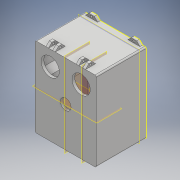
# Autodesk Inventor part: Base
Saved by Autodesk Inventor 2017 (Build 210142000, 142)
## iProperties
Created: 2017-05-28
Part Number: Base
Material: Generic
Document SubType Name: Modeling
Designer: William
Density: 1 g/cm^3
Appearance: Default
Author: William
Autodesk Inventor part; units mm, degrees
ref_plane "YZ Plane" through (0, 0, 0) normal (1, 0, 0) x (0, 1, 0)
ref_plane "XZ Plane" through (0, 0, 0) normal (0, 1, 0) x (-1, 0, 0)
ref_plane "XY Plane" through (0, 0, 0) normal (0, 0, 1) x (1, 0, 0)
sketch "Sketch1" plane through (0, 0, 0) normal (0, 1, 0) x (-1, 0, 0)
  line L0 (0, 0) -> (47, 0) construction
  line L1 (47, 0) -> (47, -100) construction
  line L2 (47, -100) -> (0, -100) construction
  line L3 (0, -100) -> (0, 0) construction
  circle A0 centre (4, -4) radius 1.6 construction
  circle A1 centre (43, -4) radius 1.6 construction
  circle A2 centre (43, -96) radius 1.729 construction
  line L4 (23.5, 0) -> (23.5, -100) construction
  line L5 (23.5, -13) -> (18.5, -13) construction
  line L6 (18.5, -13) -> (0.5, -13) construction
  circle A3 centre (0.5, -13) radius 13.5 construction
  line L7 (23.5, -13) -> (46.5, -13) construction
  circle A4 centre (46.5, -13) radius 13.5 construction
  circle A5 centre (46.5, -13) radius 13.5
  circle A6 centre (0.5, -13) radius 13.5
  circle A7 centre (23.5, -50) radius 8
  line L8 (65, 5.5) -> (-18, 5.5)
  line L9 (-18, 5.5) -> (-18, -105)
  line L10 (-18, -105) -> (65, -105)
  line L11 (65, -105) -> (65, 5.5)
  dimension "d0" = 47
  dimension "d1" = 100
  dimension "d2" = 3.2
  dimension "d3" = 4
  dimension "d4" = 4
  dimension "d5" = 4
  dimension "d6" = 43
  dimension "d7" = 3.2
  dimension "d8" = 43
  dimension "d9" = 96
  dimension "d11" = 23.5
  dimension "d12" = 5
  dimension "d13" = 13
  dimension "d14" = 18
  dimension "d15" = 27
  dimension "d16" = 23
  dimension "d17" = 27
  dimension "d18" = 16
  dimension "d19" = 50
  dimension "d20" = 5
  dimension "d21" = 5
  dimension "d22" = 5
  dimension "d23" = 5
  constraints: 24 end point, 8 centre point, 4 coincident, 4 horizontal, 4 parallel, 4 perpendicular, 3 midpoint, 2 concentric, 1 point on line
  measures "d0" distance of L1.end L2.end
  measures "d1" distance of L0.end L1.end
  measures "d2" diameter of A0
  measures "d3" distance from line of L0 A0.centre
  measures "d4" distance from line of L3 A0.centre
  measures "d5" distance from line of L0 A1.centre
  measures "d6" distance from line of L3 A1.centre
  measures "d7" diameter of A1
  measures "d8" distance from line of L3 A2.centre
  measures "d9" distance from line of L0 A2.centre
  measures "d11" distance between parallel lines of L3 L4
  measures "d12" distance of L5.start L5.end
  measures "d13" distance between parallel lines of L0 L5
  measures "d14" distance of L5.end L6.end
  measures "d15" diameter of A3
  measures "d16" distance of L5.start L7.end
  measures "d17" diameter of A4
  measures "d18" diameter of A7
  measures "d19" distance of L4.start A7.centre
  measures "d20" distance edge to line of A4 L11
  measures "d21" distance edge to line of A6 L9
  measures "d22" distance edge to line of A4 L8
  measures "d23" distance between parallel lines of L2 L10
extrude "Extrusion1" add sketch "Sketch1" along normal blind 4
sketch "Sketch3" plane through (0, 0, 0) normal (0, -1, 0) x (1, 0, 0)
  line L0 (22, -109) -> (-69, -109)
  line L1 (-69, -109) -> (-69, 9.5)
  line L2 (-69, 9.5) -> (22, 9.5)
  line L3 (22, 9.5) -> (22, -109)
  line L4 (-65, 5.5) -> (18, 5.5) projected
  line L5 (18, 5.5) -> (18, -105) projected
  line L6 (-65, 5.5) -> (18, 5.5)
  line L7 (18, 5.5) -> (18, -105)
  line L8 (18, -105) -> (-65, -105)
  line L9 (-65, -105) -> (-65, 5.5)
  point P0 (0, 0)
  dimension "d30" = 4
  dimension "d31" = 4
  dimension "d32" = 4
  dimension "d33" = 4
  constraints: 16 end point, 4 parallel, 2 horizontal, 2 perpendicular
  measures "d30" distance between parallel lines of L3 L5
  measures "d31" distance between parallel lines of L2 L4
  measures "d32" distance between parallel lines of L1 L9
  measures "d33" distance between parallel lines of L0 L8
extrude "Extrusion2" add sketch "Sketch3" against normal blind 74
sketch "Sketch4" plane through (0, 74, 0) normal (0, 1, 0) x (1, 0, 0)
  line L0 (-68, -8.5) -> (21, -8.5)
  line L1 (21, -8.5) -> (21, 108)
  line L2 (21, 108) -> (-68, 108)
  line L3 (-68, 108) -> (-68, -8.5)
  line L4 (19, 106) -> (-66, 106)
  line L5 (-66, 106) -> (-66, -6.5)
  line L6 (-66, -6.5) -> (19, -6.5)
  line L7 (19, -6.5) -> (19, 106)
  line L8 (-69, -9.5) -> (22, -9.5) projected
  line L9 (22, -9.5) -> (22, 109) projected
  line L10 (22, 109) -> (-69, 109) projected
  line L11 (-69, 109) -> (-69, -9.5) projected
  point P0 (0, 0)
  dimension "d36" = 1
  dimension "d37" = 2
  dimension "d38" = 1
  dimension "d39" = 2
  dimension "d40" = 1
  dimension "d41" = 2
  dimension "d42" = 1
  dimension "d43" = 2
  constraints: 16 end point, 4 parallel, 2 horizontal, 2 perpendicular
  measures "d36" distance between parallel lines of L8 L0
  measures "d37" distance between parallel lines of L0 L6
  measures "d38" distance between parallel lines of L9 L1
  measures "d39" distance between parallel lines of L1 L7
  measures "d40" distance between parallel lines of L10 L2
  measures "d41" distance between parallel lines of L2 L4
  measures "d42" distance between parallel lines of L11 L3
  measures "d43" distance between parallel lines of L3 L5
extrude "Extrusion3" cut sketch "Sketch4" against normal blind 4 contours L3 L2 L1 L0
fillet "Fillet1" radius 2 16 edges at (-69, 37, 9.5) (-68, 72, 8.5) (-66, 72, 6.5) (-65, 39, 5.5) (19, 72, 6.5) (21, 72, 8.5) (18, 39, 5.5) (22, 37, 9.5) (22, 37, -109) (19, 72, -106) (18, 39, -105) (21, 72, -108) (-65, 39, -105) (-68, 72, -108) (-69, 37, -109) (-66, 72, -106)
ref_plane "Work Plane1" through (0, 64, 0) normal (0, 1, 0) x (1, 0, 0)
sketch "Sketch6" plane through (0, 64, 0) normal (0, 1, 0) x (1, 0, 0)
  line L0 (0, 0) -> (-47, 0) construction
  line L1 (-47, 0) -> (-47, 100) construction
  line L2 (-47, 100) -> (0, 100) construction
  line L3 (0, 100) -> (0, 0) construction
  circle A0 centre (-4, 4) radius 1.6 construction
  circle A1 centre (-42.7634, 4) radius 1.6 construction
  line L4 (18, -3.5) -> (18, 103) projected
  line L5 (10, 34.5) -> (10, 54.5)
  line L6 (16, -5.5) -> (-63, -5.5) projected
  circle A2 centre (14, 38.5) radius 1.6
  circle A3 centre (14, 50.5) radius 1.6
  line L7 (10, 34.5) -> (18, 26.5)
  line L8 (10, 34.5) -> (21.3137, 34.5) construction
  line L9 (10, 54.5) -> (18, 62.5)
  line L10 (10, 54.5) -> (21.3137, 54.5) construction
  line L11 (18, 26.5) -> (18, 62.5)
  line L12 (-57, 34.5) -> (-57, 54.5)
  line L13 (-57, 34.5) -> (-37, 34.5) construction
  line L14 (-65, 103) -> (-65, -3.5) projected
  line L15 (-57, 34.5) -> (-65, 26.5)
  line L16 (-57, 34.5) -> (-45.6863, 34.5) construction
  line L17 (-57, 54.5) -> (-65, 62.5)
  line L18 (-57, 54.5) -> (-45.6863, 54.5) construction
  line L19 (-65, 62.5) -> (-65, 26.5)
  circle A4 centre (-61, 38.5) radius 1.6
  circle A5 centre (-61, 50.5) radius 1.6
  dimension "d48" = 47
  dimension "d49" = 100
  dimension "d50" = 3.2
  dimension "d51" = 4
  dimension "d52" = 4
  dimension "d53" = 3.2
  dimension "d55" = 20
  dimension "d57" = 3.2
  dimension "d58" = 3.2
  dimension "d61" = 4
  dimension "d62" = 4
  dimension "d63" = 45
  dimension "d64" = 45
  dimension "d65" = 20
  dimension "d66" = 90
  dimension "d67" = 8
  dimension "d68" = 135
  dimension "d69" = 135
  dimension "d70" = 3.2
  dimension "d71" = 3.2
  dimension "d100" = 12
  dimension "d101" = 0
  dimension "d102" = 4
  dimension "d103" = 12
  constraints: 34 end point, 6 centre point, 6 horizontal, 5 equal length, 4 point on line, 2 collinear, 2 parallel, 1 perpendicular, 1 vertical
  measures "d48" distance of L1.end L2.end
  measures "d49" distance of L0.end L1.end
  measures "d50" diameter of A0
  measures "d51" distance from line of L3 A0.centre
  measures "d52" distance from line of L0 A0.centre
  measures "d53" diameter of A1
  measures "d55" distance of L5.start L5.end
  measures "d57" diameter of A2
  measures "d58" diameter of A3
  measures "d61" distance from line of L5 A2.centre
  measures "d62" distance from line of L5 A3.centre
  measures "d63" angle of L7 L8
  measures "d64" angle of L10 L9
  measures "d65" distance of L12.start L12.end
  measures "d66" angle of L13 L12
  measures "d67" distance between parallel lines of L14 L12
  measures "d68" angle of L15 L16
  measures "d69" angle of L18 L17
  measures "d70" diameter of A4
  measures "d71" diameter of A5
  measures "d100" distance of A4.centre A5.centre
  measures "d101" vertical distance of A3.centre A5.centre
  measures "d102" distance from line of L8 A2.centre
  measures "d103" distance of A2.centre A3.centre
extrude "Extrusion4" add sketch "Sketch6" against normal up to next
sketch "Sketch8" plane through (0, 74, 0) normal (0, 1, 0) x (1, 0, 0)
  line L0 (-51, -14.5) -> (-59, -14.5)
  line L1 (-69, 107) -> (-69, -7.5) projected
  line L2 (4, -14.5) -> (12, -14.5)
  line L3 (22, -7.5) -> (22, 107) projected
  line L4 (-59, -14.5) -> (-64, -9.5)
  line L5 (-59, -14.5) -> (-51.9289, -14.5) construction
  line L6 (-51, -14.5) -> (-46, -9.5)
  line L7 (-51, -14.5) -> (-43.9289, -14.5) construction
  line L8 (-46, -9.5) -> (-64, -9.5)
  line L9 (-67, -9.5) -> (20, -9.5) projected
  line L10 (4, -14.5) -> (-1, -9.5)
  line L11 (4, -14.5) -> (11.0711, -14.5) construction
  line L12 (12, -14.5) -> (17, -9.5)
  line L13 (12, -14.5) -> (19.0711, -14.5) construction
  line L14 (17, -9.5) -> (-1, -9.5)
  circle A0 centre (-55.4645, -12) radius 1.6
  circle A1 centre (8, -12) radius 1.6
  line L15 (20, 109) -> (-67, 109) projected
  line L16 (-51, 114) -> (-59, 114)
  line L17 (4, 114) -> (12, 114)
  line L18 (-51, 114) -> (-46, 109)
  line L19 (-51, 114) -> (-43.9289, 114) construction
  line L20 (-59, 114) -> (-64, 109)
  line L21 (-59, 114) -> (-51.9289, 114) construction
  line L22 (-64, 109) -> (-46, 109)
  line L23 (4, 114) -> (-1, 109)
  line L24 (4, 114) -> (11.0711, 114) construction
  line L25 (12, 114) -> (17, 109)
  line L26 (-1, 109) -> (17, 109)
  circle A2 centre (-55, 111.5) radius 1.6
  circle A3 centre (8, 111.5) radius 1.6
  point P0 (0, 0)
  dimension "d74" = 8
  dimension "d77" = 8
  dimension "d80" = 135
  dimension "d81" = 45
  dimension "d82" = 135
  dimension "d83" = 45
  dimension "d84" = 3.2
  dimension "d85" = 3.2
  dimension "d86" = 8
  dimension "d89" = 8
  dimension "d91" = 10
  dimension "d92" = 10
  dimension "d93" = 45
  dimension "d94" = 135
  dimension "d95" = 135
  dimension "d96" = 3.2
  dimension "d97" = 3.2
  constraints: 46 end point, 7 equal length, 7 horizontal, 6 point on line, 4 centre point, 4 collinear
  measures "d74" distance of L0.start L0.end
  measures "d77" distance of L2.end L2.start
  measures "d80" angle of L5 L4
  measures "d81" angle of L7 L6
  measures "d82" angle of L11 L10
  measures "d83" angle of L13 L12
  measures "d84" diameter of A0
  measures "d85" diameter of A1
  measures "d86" distance of L16.end L16.start
  measures "d89" distance of L17.start L17.end
  measures "d91" distance from line of L3 L17.end
  measures "d92" distance from line of L1 L16.end
  measures "d93" angle of L18 L19
  measures "d94" angle of L20 L21
  measures "d95" angle of L23 L24
  measures "d96" diameter of A2
  measures "d97" diameter of A3
extrude "Extrusion5" add sketch "Sketch8" against normal blind 4
sketch "Sketch9" plane through (0, 74, 0) normal (0, 1, 0) x (1, 0, 0)
  circle A0 centre (-55, 111.5) radius 1.6 projected
  circle A1 centre (-55.4645, -12) radius 1.6 projected
  circle A2 centre (8, -12) radius 1.6 projected
  circle A3 centre (8, 111.5) radius 1.6 projected
  arc A4 (-67, 109) -> (-69, 107) centre (-67, 107) ccw projected
  line L0 (-69, 107) -> (-69, -7.5) projected
  arc A5 (-69, -7.5) -> (-67, -9.5) centre (-67, -7.5) ccw projected
  line L1 (-67, -9.5) -> (-64, -9.5) projected
  line L2 (-59, -14.5) -> (-64, -9.5) projected
  line L3 (-51, -14.5) -> (-59, -14.5) projected
  line L4 (-46, -9.5) -> (-51, -14.5) projected
  line L5 (-46, -9.5) -> (-1, -9.5) projected
  line L6 (-1, -9.5) -> (4, -14.5) projected
  line L7 (4, -14.5) -> (12, -14.5) projected
  line L8 (12, -14.5) -> (17, -9.5) projected
  line L9 (17, -9.5) -> (20, -9.5) projected
  arc A6 (20, -9.5) -> (22, -7.5) centre (20, -7.5) ccw projected
  line L10 (22, -7.5) -> (22, 107) projected
  arc A7 (22, 107) -> (20, 109) centre (20, 107) ccw projected
  line L11 (20, 109) -> (17, 109) projected
  line L12 (17, 109) -> (12, 114) projected
  line L13 (12, 114) -> (4, 114) projected
  line L14 (4, 114) -> (-1, 109) projected
  line L15 (-1, 109) -> (-46, 109) projected
  line L16 (-46, 109) -> (-51, 114) projected
  line L17 (-51, 114) -> (-59, 114) projected
  line L18 (-59, 114) -> (-64, 109) projected
  line L19 (-64, 109) -> (-67, 109) projected
  line L20 (21, 106) -> (21, -6.5) projected
  arc A8 (19, -8.5) -> (21, -6.5) centre (19, -6.5) ccw projected
  line L21 (19, -8.5) -> (-66, -8.5) projected
  arc A9 (-68, -6.5) -> (-66, -8.5) centre (-66, -6.5) ccw projected
  line L22 (-68, -6.5) -> (-68, 106) projected
  arc A10 (-66, 108) -> (-68, 106) centre (-66, 106) ccw projected
  line L23 (-66, 108) -> (19, 108) projected
  arc A11 (21, 106) -> (19, 108) centre (19, 106) ccw projected
  point P0 (0, 0)
ref_plane "Work Plane2" through (2, 0, 7.5) normal (1, 0, 0) x (0, 0, -1)
sketch "Sketch10" plane through (2, 0, 7.5) normal (1, 0, 0) x (0, 0, -1)
  line L0 (-7, 5) -> (-7, 10)
  line L1 (0, 0) -> (114.5, 0) projected
  line L2 (-7, 5) -> (-2, 0)
  line L3 (-7, 10) -> (-2, 15)
  line L4 (-2, 15) -> (-2, 0)
  line L5 (0, 74) -> (0, 0) projected
  circle A0 centre (-4.5, 7.5) radius 1.6
  point P0 (7.5, 0)
  dimension "d106" = 5
  dimension "d108" = 3.2
  constraints: 8 end point, 1 centre point, 1 parallel, 1 perpendicular
  measures "d106" distance of L0.start L0.end
  measures "d108" diameter of A0
extrude "Extrusion6" add sketch "Sketch10" along normal blind 4
ref_plane "Work Plane3" through (-23.5, 0, 7.5) normal (1, 0, 0) x (0, 0, -1)
ref_plane "Work Plane5" through (20, 0, -49.75) normal (0, 0, 1) x (1, 0, 0)
pattern_linear "Rectangular Pattern1" count 2 spacing 10 along (-1, 0, 0) of "Extrusion6"
mirror "Mirror3" about plane through (-23.5, 0, 7.5) normal (1, 0, 0) of "Extrusion6", "Rectangular Pattern1"
mirror "Mirror4" about plane through (20, 0, -49.75) normal (0, 0, 1) of "Extrusion6", "Rectangular Pattern1", "Mirror3"
body "Solid1"
